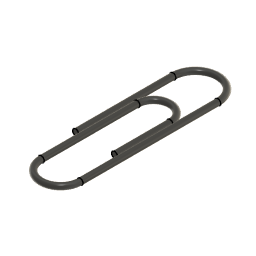
Paper_Clip (Autodesk Fusion 360 design; units mm, degrees)
Autodesk Fusion 360 part; units mm, degrees
sketch "Sketch1" plane through (0, 0, 0) normal (0, 0, 1) x (1, 0, 0)
  line L0 (0, 0) -> (0, 16.25)
  line L1 (7.5, 16.25) -> (7.5, -6.75)
  line L2 (1, -6.75) -> (1, 9.25)
  arc A0 (3.75, 20) -> (0, 16.25) centre (3.75, 16.25) ccw
  arc A1 (7.5, 16.25) -> (3.75, 20) centre (3.75, 16.25) ccw
  arc A2 (4.25, -10) -> (7.5, -6.75) centre (4.25, -6.75) ccw
  arc A3 (1, -6.75) -> (4.25, -10) centre (4.25, -6.75) ccw
  line L3 (6.5, 9.25) -> (6.5, 0)
  arc A4 (3.75, 12) -> (1, 9.25) centre (3.75, 9.25) ccw
  arc A5 (6.5, 9.25) -> (3.75, 12) centre (3.75, 9.25) ccw
  point P0 (0, 20)
  point P1 (7.5, 20)
  point P2 (7.5, -10)
  point P3 (1, -10)
  point P4 (1, 12)
  point P5 (6.5, 12)
  dimension "d1" = 20
  dimension "d2" = 7.5
  dimension "d4" = 30
  dimension "d5" = 6.5
  dimension "d6" = 22
  dimension "d7" = 5.5
  dimension "d8" = 3.75
  dimension "d9" = 3.25
  dimension "d10" = 12
  dimension "d11" = 2.75
  constraint vertical L0
  constraint coincident L0.start origin
  constraint coincident P0 L0
  constraint tangent L0 A0
  constraint coincident P1 L1
  constraint tangent L1 A1
  constraint equal A0 A1
  constraint coincident A0.start A1.end
  constraint vertical L1
  constraint coincident P2 L1
  constraint tangent L1 A2
  constraint coincident P3 L2
  constraint tangent L2 A3
  constraint equal A2 A3
  constraint coincident A2.start A3.end
  constraint vertical L2
  constraint coincident P4 L2
  constraint tangent L2 A4
  constraint coincident P5 L3
  constraint tangent L3 A5
  constraint equal A4 A5
  constraint coincident A4.start A5.end
  measures "d1" distance of L0.start P0
  measures "d2" distance of P0 P1
  measures "d4" distance of P1 P2
  measures "d5" distance of P2 P3
  measures "d6" distance of P3 P4
  measures "d7" distance of P4 P5
  measures "d8" radius of A0
  measures "d9" radius of A2
  measures "d10" distance of P5 L3.end
  measures "d11" radius of A4
sketch "Sketch4" plane through (0, 0, 0) normal (0, 1, 0) x (1, 0, 0)
  circle A0 centre (0, 0) radius 0.5
  dimension "d12" = 1
  constraint coincident A0.centre origin
  measures "d12" diameter of A0
sweep "Sweep1" add profiles "Sketch4" path "Sketch1" along L3 A5 A4 L2 A3 A2 L1 A1 A0 L0 section 1
